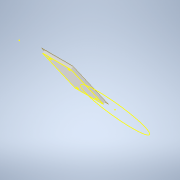
# Autodesk Inventor part: shooter spacer
Saved by Autodesk Inventor 2021 (Build 250183000, 183)
## iProperties
Created: 2021-04-02
Part Number: shooter spacer
Material: Generic
Document SubType Name: Modeling
Designer: deli
Density: 1 g/cm^3
Appearance: Default
Author: deli
Autodesk Inventor part; units mm, degrees
ref_plane "YZ Plane" through (0, 0, 0) normal (1, 0, 0) x (0, 1, 0)
ref_plane "XZ Plane" through (0, 0, 0) normal (0, 1, 0) x (-1, 0, 0)
ref_plane "XY Plane" through (0, 0, 0) normal (0, 0, 1) x (1, 0, 0)
ref_plane "Work Plane1" through (87.3148, -183.736, 102.4116) normal (0, -0.5735764, 0.819152) x (0, 0.819152, 0.5735764)
sketch "Sketch1" plane through (87.3148, -183.736, 102.4116) normal (0, -0.5735764, 0.819152) x (0, 0.819152, 0.5735764)
  line L0 (96, -2.5) -> (96, 45.5) projected
  line L1 (0, 45.5) -> (96, 45.5) projected
  line L2 (0, -2.5) -> (0, 45.5) projected
  line L3 (-64, -2.5) -> (104, -2.5) projected
  circle A0 centre (8, -26.5) radius 50.8 projected
  circle A1 centre (88, 37.5) radius 2 projected
  arc A2 (88.9632, 3.7472) -> (86.3648, 4.3484) centre (88, 5.5) ccw projected
  circle A3 centre (8, 37.5) radius 2 projected
  circle A4 centre (8, 5.5) radius 2 projected
  circle A5 centre (88, 5.5) radius 2
  circle A6 centre (8, -26.5) radius 52.8
  point P0 (91.7668, 87.3148)
  point P1 (88.9632, 3.7472)
  point P2 (86.3648, 4.3484)
  dimension "d0" = 4
  dimension "d1" = 2
  constraints: 2 centre point, 1 coincident
  measures "d0" diameter of A5
  measures "d1" radial gap between concentric circles of A0 A6
extrude "Extrusion1" add sketch "Sketch1" along normal blind 4 contours L3 A6 L2 L1 L0 | L3 A0 L2 A6 | L3 L2 A0 picked at (50.2151, 2.6583) picked at (20.4941, -0.4567)
sketch "Sketch2" plane through (87.3148, -186.0303, 105.6882) normal (0, -0.5735764, 0.819152) x (1, 0, 0)
  line L0 (-45.5, 0) -> (2.5, 0) projected
  line L1 (2.5, 0) -> (2.5, 96) projected
  line L2 (2.5, 96) -> (-45.5, 96) projected
  line L3 (-45.5, 96) -> (-45.5, 0) projected
  circle A0 centre (-5.5, 8) radius 2 projected
  circle A1 centre (-37.5, 8) radius 2 projected
  circle A2 centre (-5.5, 88) radius 2 projected
  circle A3 centre (-37.5, 88) radius 2 projected
  circle A4 centre (26.5, 8) radius 50.8 projected
  circle A5 centre (26.5, 8) radius 54.8
  point P0 (-87.3148, 91.7668)
  point P1 (-27.7129, 0)
  point P2 (2.5, 57.265)
  dimension "d4" = 4
  constraints: 1 centre point
  measures "d4" radial gap between concentric circles of A4 A5
extrude "Extrusion2" add sketch "Sketch2" against normal blind 9.398 contours L3 L2 L1 A5 L0
body "Solid1"
